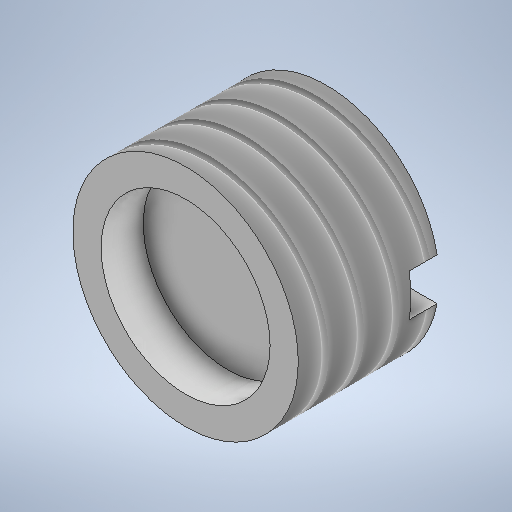
# Autodesk Inventor part: 138
Saved by Autodesk Inventor 2025.1 (Build 291241000, 241)
## iProperties
Created: 2024-08-05
Part Number: 138
Material: Generisch
Document SubType Name: Modeling
Designer: ffogue
Density: 1 g/cm^3
Appearance: Vorgabe
Author: ffogue
Autodesk Inventor part; units mm, degrees
ref_plane "YZ Plane" through (0, 0, 0) normal (1, 0, 0) x (0, 1, 0)
ref_plane "XZ Plane" through (0, 0, 0) normal (0, 1, 0) x (-1, 0, 0)
ref_plane "XY Plane" through (0, 0, 0) normal (0, 0, 1) x (1, 0, 0)
sketch "Sketch1" plane through (0, 0, 0) normal (0, 0, 1) x (1, 0, 0)
  line L0 (0, 0) -> (4, 0)
  line L1 (4, 0) -> (4, 5)
  line L2 (4, 5) -> (0, 5)
  line L3 (0, 5) -> (0, 0)
  point P0 (0, 2.5)
  dimension "d0" = 5
  dimension "d1" = 8
  constraints: 8 end point, 3 perpendicular, 1 horizontal, 1 midpoint
  measures "d0" distance between parallel lines of L0 L2
  measures "d1" diameter of L1 point (0, 2.5)
revolve "Revolution1" add sketch "Sketch1" angle 360 about axis through (0, 5, 0) along (0, -1, 0)
sketch "Sketch2" plane through (0, 5, 0) normal (0, 1, 0) x (1, 0, 0)
  circle A0 centre (0, 0) radius 4 projected
  circle A1 centre (0, 0) radius 4 projected
  line L0 (-3.9291, -0.75) -> (3.9291, -0.75)
  line L1 (-3.9291, 0.75) -> (3.9291, 0.75)
  point P0 (0, -0.75)
  dimension "d3" = 0.75
  dimension "d4" = 0.75
  constraints: 4 end point, 4 point on circle, 1 horizontal, 1 midpoint, 1 parallel
  measures "d3" distance of point (0, 0) point (0, -0.75)
  measures "d4" distance from line of L1 point (0, 0)
extrude "Extrusion1" cut sketch "Sketch2" against normal blind 1 contours A0 L0 L1
sketch "Sketch3" plane through (0, 0, 0) normal (0, -1, 0) x (1, 0, 0)
  circle A0 centre (0, 0) radius 4 projected
  constraints: 1 coincident
hole "Hole1" at (0, 0, 0) direction (0, 1, 0) diameter 6 depth 1.5
thread "Thread1" size "M8x1.25" class "6g" standard "ISO Metric profile" length 10
equation "\"d4\" = d3"
body "Solid1"
